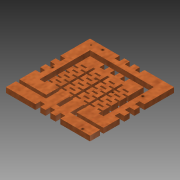
# Autodesk Inventor part: mech
Saved by Autodesk Inventor 2014 SP1 (Build 180222100, 222)
## iProperties
Created: 2015-02-17
Part Number: mech
Material: Wood (Cherry)
Document SubType Name: Modeling
Designer: Erin
Density: 0.63 g/cm^3
Appearance: Cherry - Natural Low Gloss
Author: Erin
Autodesk Inventor part; units mm, degrees
ref_plane "YZ Plane" through (0, 0, 0) normal (1, 0, 0) x (0, 1, 0)
ref_plane "XZ Plane" through (0, 0, 0) normal (0, 1, 0) x (-1, 0, 0)
ref_plane "XY Plane" through (0, 0, 0) normal (0, 0, 1) x (1, 0, 0)
sketch "slots" plane through (0, 0, 0) normal (0, 0, 1) x (1, 0, 0)
  line L0 (61.2067, 31.1821) -> (64.2567, 31.1821)
  line L1 (64.2567, 31.1821) -> (64.2567, 28.1071)
  line L2 (64.2567, 28.1071) -> (61.2067, 28.1071)
  line L3 (61.2067, 28.1071) -> (61.2067, 31.1821)
  line L4 (68.9317, 33.8834) -> (68.9317, 26.9198) construction
  line L5 (67.4067, 31.1821) -> (70.4567, 31.1821)
  line L6 (70.4567, 31.1821) -> (70.4567, 28.1071)
  line L7 (70.4567, 28.1071) -> (67.4067, 28.1071)
  line L8 (67.4067, 28.1071) -> (67.4067, 31.1821)
  line L9 (73.6067, 31.1821) -> (76.6567, 31.1821)
  line L10 (76.6567, 31.1821) -> (76.6567, 28.1071)
  line L11 (76.6567, 28.1071) -> (73.6067, 28.1071)
  line L12 (73.6067, 28.1071) -> (73.6067, 31.1821)
  line L13 (68.9317, 28.1071) -> (68.9317, 27.1937) construction
  point P0 (68.8645, 30.3856)
  dimension "d2" = 3.05
  dimension "d3" = 3.075
  dimension "d99" = 3.15
  dimension "d100" = 3.15
  measures "d2" distance of L1.end L2.end
  measures "d3" distance of L0.end L1.end
  measures "d99" distance between parallel lines of L8 L1
  measures "d100" distance between parallel lines of L12 L6
sketch "flexure" plane through (0, 0, 0) normal (0, 0, 1) x (1, 0, 0)
  line L0 (48.9032, 41.5133) -> (55.9032, 41.5133)
  line L1 (55.9032, 41.5133) -> (55.9032, 19.5133)
  line L2 (55.9032, 19.5133) -> (48.9032, 19.5133)
  line L3 (48.9032, 19.5133) -> (48.9032, 41.5133)
  line L4 (48.9032, 32.2633) -> (51.4486, 32.2633)
  line L5 (51.4486, 32.2633) -> (51.4486, 31.2633)
  line L6 (51.4486, 31.2633) -> (48.9032, 31.2633)
  line L7 (48.9032, 31.2633) -> (48.9032, 32.2633)
  line L8 (53.3577, 31.2633) -> (53.3577, 32.2633)
  line L9 (55.9032, 31.2633) -> (53.3577, 31.2633)
  line L10 (53.3577, 32.2633) -> (55.9032, 32.2633)
  line L11 (55.9032, 32.2633) -> (55.9032, 31.2633)
  line L12 (50.8123, 29.7633) -> (53.9941, 29.7633)
  line L13 (53.9941, 29.7633) -> (53.9941, 28.7633)
  line L14 (53.9941, 28.7633) -> (50.8123, 28.7633)
  line L15 (50.8123, 28.7633) -> (50.8123, 29.7633)
  line L16 (48.9032, 30.5133) -> (55.9032, 30.5133) construction
  line L17 (55.9032, 30.5133) -> (48.9032, 30.5133) construction
  line L18 (53.3577, 27.2633) -> (55.9032, 27.2633)
  line L19 (55.9032, 27.2633) -> (55.9032, 26.2633)
  line L20 (55.9032, 26.2633) -> (53.3577, 26.2633)
  line L21 (53.3577, 26.2633) -> (53.3577, 27.2633)
  line L22 (50.8123, 24.7633) -> (53.9941, 24.7633)
  line L23 (53.9941, 24.7633) -> (53.9941, 23.7633)
  line L24 (53.9941, 23.7633) -> (50.8123, 23.7633)
  line L25 (50.8123, 23.7633) -> (50.8123, 24.7633)
  line L26 (48.9032, 27.2633) -> (51.4486, 27.2633)
  line L27 (51.4486, 27.2633) -> (51.4486, 26.2633)
  line L28 (51.4486, 26.2633) -> (48.9032, 26.2633)
  line L29 (48.9032, 26.2633) -> (48.9032, 27.2633)
  line L30 (48.9032, 25.5133) -> (55.9032, 25.5133) construction
  line L31 (55.9032, 25.5133) -> (48.9032, 25.5133) construction
  line L32 (53.3577, 37.2633) -> (55.9032, 37.2633)
  line L33 (55.9032, 37.2633) -> (55.9032, 36.2633)
  line L34 (55.9032, 36.2633) -> (53.3577, 36.2633)
  line L35 (53.3577, 36.2633) -> (53.3577, 37.2633)
  line L36 (50.8123, 34.7633) -> (53.9941, 34.7633)
  line L37 (53.9941, 34.7633) -> (53.9941, 33.7633)
  line L38 (53.9941, 33.7633) -> (50.8123, 33.7633)
  line L39 (50.8123, 33.7633) -> (50.8123, 34.7633)
  line L40 (48.9032, 37.2633) -> (51.4486, 37.2633)
  line L41 (51.4486, 37.2633) -> (51.4486, 36.2633)
  line L42 (51.4486, 36.2633) -> (48.9032, 36.2633)
  line L43 (48.9032, 36.2633) -> (48.9032, 37.2633)
  line L44 (48.9032, 35.5133) -> (55.9032, 35.5133) construction
  line L45 (55.9032, 35.5133) -> (48.9032, 35.5133) construction
  line L46 (53.3577, 32.2633) -> (55.9032, 32.2633)
  line L47 (55.9032, 32.2633) -> (55.9032, 31.2633)
  line L48 (55.9032, 31.2633) -> (53.3577, 31.2633)
  line L49 (53.3577, 31.2633) -> (53.3577, 32.2633)
  line L50 (50.8123, 29.7633) -> (53.9941, 29.7633)
  line L51 (53.9941, 29.7633) -> (53.9941, 28.7633)
  line L52 (53.9941, 28.7633) -> (50.8123, 28.7633)
  line L53 (50.8123, 28.7633) -> (50.8123, 29.7633)
  line L54 (48.9032, 32.2633) -> (51.4486, 32.2633)
  line L55 (51.4486, 32.2633) -> (51.4486, 31.2633)
  line L56 (51.4486, 31.2633) -> (48.9032, 31.2633)
  line L57 (48.9032, 31.2633) -> (48.9032, 32.2633)
  line L58 (48.9032, 30.5133) -> (55.9032, 30.5133) construction
  line L59 (55.9032, 30.5133) -> (48.9032, 30.5133) construction
  line L60 (53.3577, 22.2633) -> (55.9032, 22.2633)
  line L61 (55.9032, 22.2633) -> (55.9032, 21.2633)
  line L62 (55.9032, 21.2633) -> (53.3577, 21.2633)
  line L63 (53.3577, 21.2633) -> (53.3577, 22.2633)
  line L64 (50.8123, 19.7633) -> (53.9941, 19.7633)
  line L65 (53.9941, 19.7633) -> (53.9941, 18.7633)
  line L66 (53.9941, 18.7633) -> (50.8123, 18.7633)
  line L67 (50.8123, 18.7633) -> (50.8123, 19.7633)
  line L68 (48.9032, 22.2633) -> (51.4486, 22.2633)
  line L69 (51.4486, 22.2633) -> (51.4486, 21.2633)
  line L70 (51.4486, 21.2633) -> (48.9032, 21.2633)
  line L71 (48.9032, 21.2633) -> (48.9032, 22.2633)
  line L72 (48.9032, 20.5133) -> (55.9032, 20.5133) construction
  line L73 (55.9032, 20.5133) -> (48.9032, 20.5133) construction
  line L74 (53.3577, 27.2633) -> (55.9032, 27.2633)
  line L75 (55.9032, 27.2633) -> (55.9032, 26.2633)
  line L76 (55.9032, 26.2633) -> (53.3577, 26.2633)
  line L77 (53.3577, 26.2633) -> (53.3577, 27.2633)
  line L78 (50.8123, 24.7633) -> (53.9941, 24.7633)
  line L79 (53.9941, 24.7633) -> (53.9941, 23.7633)
  line L80 (53.9941, 23.7633) -> (50.8123, 23.7633)
  line L81 (50.8123, 23.7633) -> (50.8123, 24.7633)
  line L82 (48.9032, 27.2633) -> (51.4486, 27.2633)
  line L83 (51.4486, 27.2633) -> (51.4486, 26.2633)
  line L84 (51.4486, 26.2633) -> (48.9032, 26.2633)
  line L85 (48.9032, 26.2633) -> (48.9032, 27.2633)
  line L86 (48.9032, 25.5133) -> (55.9032, 25.5133) construction
  line L87 (55.9032, 25.5133) -> (48.9032, 25.5133) construction
  line L88 (53.3577, 42.2633) -> (55.9032, 42.2633)
  line L89 (55.9032, 42.2633) -> (55.9032, 41.2633)
  line L90 (55.9032, 41.2633) -> (53.3577, 41.2633)
  line L91 (53.3577, 41.2633) -> (53.3577, 42.2633)
  line L92 (50.8123, 39.7633) -> (53.9941, 39.7633)
  line L93 (53.9941, 39.7633) -> (53.9941, 38.7633)
  line L94 (53.9941, 38.7633) -> (50.8123, 38.7633)
  line L95 (50.8123, 38.7633) -> (50.8123, 39.7633)
  line L96 (48.9032, 42.2633) -> (51.4486, 42.2633)
  line L97 (51.4486, 42.2633) -> (51.4486, 41.2633)
  line L98 (51.4486, 41.2633) -> (48.9032, 41.2633)
  line L99 (48.9032, 41.2633) -> (48.9032, 42.2633)
  line L100 (48.9032, 40.5133) -> (55.9032, 40.5133) construction
  line L101 (55.9032, 40.5133) -> (48.9032, 40.5133) construction
  line L102 (53.3577, 37.2633) -> (55.9032, 37.2633)
  line L103 (55.9032, 37.2633) -> (55.9032, 36.2633)
  line L104 (55.9032, 36.2633) -> (53.3577, 36.2633)
  line L105 (53.3577, 36.2633) -> (53.3577, 37.2633)
  line L106 (50.8123, 34.7633) -> (53.9941, 34.7633)
  line L107 (53.9941, 34.7633) -> (53.9941, 33.7633)
  line L108 (53.9941, 33.7633) -> (50.8123, 33.7633)
  line L109 (50.8123, 33.7633) -> (50.8123, 34.7633)
  line L110 (48.9032, 37.2633) -> (51.4486, 37.2633)
  line L111 (51.4486, 37.2633) -> (51.4486, 36.2633)
  line L112 (51.4486, 36.2633) -> (48.9032, 36.2633)
  line L113 (48.9032, 36.2633) -> (48.9032, 37.2633)
  line L114 (48.9032, 35.5133) -> (55.9032, 35.5133) construction
  line L115 (55.9032, 35.5133) -> (48.9032, 35.5133) construction
  line L116 (53.3577, 32.2633) -> (55.9032, 32.2633)
  line L117 (55.9032, 32.2633) -> (55.9032, 31.2633)
  line L118 (55.9032, 31.2633) -> (53.3577, 31.2633)
  line L119 (53.3577, 31.2633) -> (53.3577, 32.2633)
  line L120 (50.8123, 29.7633) -> (53.9941, 29.7633)
  line L121 (53.9941, 29.7633) -> (53.9941, 28.7633)
  line L122 (53.9941, 28.7633) -> (50.8123, 28.7633)
  line L123 (50.8123, 28.7633) -> (50.8123, 29.7633)
  line L124 (48.9032, 32.2633) -> (51.4486, 32.2633)
  line L125 (51.4486, 32.2633) -> (51.4486, 31.2633)
  line L126 (51.4486, 31.2633) -> (48.9032, 31.2633)
  line L127 (48.9032, 31.2633) -> (48.9032, 32.2633)
  line L128 (48.9032, 30.5133) -> (55.9032, 30.5133) construction
  line L129 (55.9032, 30.5133) -> (48.9032, 30.5133) construction
  point P0 (52.8239, 25.8216)
  dimension "d22" = 7
  dimension "d24" = 2.5455
  dimension "d27" = 4.4546
  dimension "d32" = 1.9091
  dimension "d33" = 3.1818
  dimension "d41" = 1
  dimension "d42" = 1
  dimension "d43" = 1.5
  dimension "d93" = 22
  dimension "d106" = 5
  dimension "d109" = 5
  dimension "d115" = 11.75
  measures "d22" distance of L1.end L2.end
  measures "d24" distance of L4.start L4.end
  measures "d27" distance of L6.end L9.end
  measures "d32" distance between parallel lines of L15 L3
  measures "d33" distance of L12.start L12.end
  measures "d41" distance of L4.end L5.end
  measures "d42" distance of L12.end L13.end
  measures "d43" distance between parallel lines of L12 L6
  measures "d93" distance of L0.end L1.end
  measures "d106" distance of L10.start L18.start
  measures "d109" distance of L10.start L32.start
  measures "d115" distance between parallel lines of L12 L0
sketch "Sketch1" plane through (0, 0, 0) normal (0, 0, 1) x (1, 0, 0)
  line L0 (-25, 25) -> (25, 25) construction
  line L1 (25, 25) -> (25, -25) construction
  line L2 (25, -25) -> (-25, -25) construction
  line L3 (-25, -25) -> (-25, 25) construction
  line L4 (-25, -25) -> (25, -25)
  line L5 (25, -25) -> (25, -19)
  line L6 (25, -19) -> (-25, -19)
  line L7 (-25, -19) -> (-25, -25)
  line L8 (0, 33.5916) -> (0, -39.9789) construction
  line L9 (-35.9054, 0) -> (42.6007, 0) construction
  line L10 (-25, 25) -> (25, 25)
  line L11 (25, 25) -> (25, 19)
  line L12 (25, 19) -> (-25, 19)
  line L13 (-25, 19) -> (-25, 25)
  line L14 (-25, 19) -> (-19, 19)
  line L15 (-19, 19) -> (-19, -17)
  line L16 (-19, -17) -> (-25, -17)
  line L17 (-25, -17) -> (-25, 19)
  line L18 (-19, -17) -> (-9, -17)
  line L19 (-9, -17) -> (-9, -11)
  line L20 (-9, -11) -> (-19, -11)
  line L21 (-19, -11) -> (-19, -17)
  line L22 (25, 19) -> (19, 19)
  line L23 (19, 19) -> (19, -17)
  line L24 (19, -17) -> (25, -17)
  line L25 (25, -17) -> (25, 19)
  line L26 (19, -17) -> (9, -17)
  line L27 (9, -17) -> (9, -11)
  line L28 (9, -11) -> (19, -11)
  line L29 (19, -11) -> (19, -17)
  line L30 (-16, 16) -> (16, 16)
  line L31 (16, 16) -> (16, 11)
  line L32 (16, 11) -> (-16, 11)
  line L33 (-16, 11) -> (-16, 16)
  line L34 (-7.2, -11) -> (-1.2, -11)
  line L35 (-1.2, -11) -> (-1.2, -19)
  line L36 (-1.2, -19) -> (-7.2, -19)
  line L37 (-7.2, -19) -> (-7.2, -11)
  line L38 (1.2, -11) -> (7.2, -11)
  line L39 (7.2, -11) -> (7.2, -19)
  line L40 (7.2, -19) -> (1.2, -19)
  line L41 (1.2, -19) -> (1.2, -11)
  line L42 (-68.1542, 16.5688) -> (-29.44, 16.5688) construction
  line L43 (-29.44, 16.5688) -> (-29.44, -5.0786) construction
  line L44 (-29.44, -5.0786) -> (-68.1542, -5.0786) construction
  line L45 (-68.1542, -5.0786) -> (-68.1542, 16.5688) construction
  circle A0 centre (-21.2866, 22) radius 0.5
  line L46 (-7.725, 25) -> (-4.675, 25)
  line L47 (-4.675, 25) -> (-4.675, 21.925)
  line L48 (-4.675, 21.925) -> (-7.725, 21.925)
  line L49 (-7.725, 21.925) -> (-7.725, 25)
  line L50 (0, 27.7013) -> (0, 20.7377) construction
  line L51 (-1.525, 25) -> (1.525, 25)
  line L52 (1.525, 25) -> (1.525, 21.925)
  line L53 (1.525, 21.925) -> (-1.525, 21.925)
  line L54 (-1.525, 21.925) -> (-1.525, 25)
  line L55 (4.675, 25) -> (7.725, 25)
  line L56 (7.725, 25) -> (7.725, 21.925)
  line L57 (7.725, 21.925) -> (4.675, 21.925)
  line L58 (4.675, 21.925) -> (4.675, 25)
  line L59 (0, 21.925) -> (0, 21.0116) construction
  line L60 (-7.725, -21.925) -> (-4.675, -21.925)
  line L61 (-4.675, -21.925) -> (-4.675, -25)
  line L62 (-4.675, -25) -> (-7.725, -25)
  line L63 (-7.725, -25) -> (-7.725, -21.925)
  line L64 (0, -19.2237) -> (0, -26.1873) construction
  line L65 (-1.525, -21.925) -> (1.525, -21.925)
  line L66 (1.525, -21.925) -> (1.525, -25)
  line L67 (1.525, -25) -> (-1.525, -25)
  line L68 (-1.525, -25) -> (-1.525, -21.925)
  line L69 (4.675, -21.925) -> (7.725, -21.925)
  line L70 (7.725, -21.925) -> (7.725, -25)
  line L71 (7.725, -25) -> (4.675, -25)
  line L72 (4.675, -25) -> (4.675, -21.925)
  line L73 (0, -25) -> (0, -25.9134) construction
  line L74 (-25, -7.725) -> (-25, -4.675)
  line L75 (-25, -4.675) -> (-21.925, -4.675)
  line L76 (-21.925, -4.675) -> (-21.925, -7.725)
  line L77 (-21.925, -7.725) -> (-25, -7.725)
  line L78 (-27.7013, 0) -> (-20.7377, 0) construction
  line L79 (-25, -1.525) -> (-25, 1.525)
  line L80 (-25, 1.525) -> (-21.925, 1.525)
  line L81 (-21.925, 1.525) -> (-21.925, -1.525)
  line L82 (-21.925, -1.525) -> (-25, -1.525)
  line L83 (-25, 4.675) -> (-25, 7.725)
  line L84 (-25, 7.725) -> (-21.925, 7.725)
  line L85 (-21.925, 7.725) -> (-21.925, 4.675)
  line L86 (-21.925, 4.675) -> (-25, 4.675)
  line L87 (-21.925, 0) -> (-21.0116, 0) construction
  line L88 (21.925, -7.725) -> (21.925, -4.675)
  line L89 (21.925, -4.675) -> (25, -4.675)
  line L90 (25, -4.675) -> (25, -7.725)
  line L91 (25, -7.725) -> (21.925, -7.725)
  line L92 (19.2237, 0) -> (26.1873, 0) construction
  line L93 (21.925, -1.525) -> (21.925, 1.525)
  line L94 (21.925, 1.525) -> (25, 1.525)
  line L95 (25, 1.525) -> (25, -1.525)
  line L96 (25, -1.525) -> (21.925, -1.525)
  line L97 (21.925, 4.675) -> (21.925, 7.725)
  line L98 (21.925, 7.725) -> (25, 7.725)
  line L99 (25, 7.725) -> (25, 4.675)
  line L100 (25, 4.675) -> (21.925, 4.675)
  line L101 (25, 0) -> (25.9134, 0) construction
  line L102 (-16, 11) -> (-9, 11)
  line L103 (-9, 11) -> (-9, -11)
  line L104 (-9, -11) -> (-16, -11)
  line L105 (-16, -11) -> (-16, 11)
  line L106 (-16, 1.75) -> (-13.4545, 1.75)
  line L107 (-13.4545, 1.75) -> (-13.4545, 0.75)
  line L108 (-13.4545, 0.75) -> (-16, 0.75)
  line L109 (-16, 0.75) -> (-16, 1.75)
  line L110 (-11.5455, 0.75) -> (-11.5455, 1.75)
  line L111 (-9, 0.75) -> (-11.5455, 0.75)
  line L112 (-11.5455, 1.75) -> (-9, 1.75)
  line L113 (-9, 1.75) -> (-9, 0.75)
  line L114 (-14.0909, -0.75) -> (-10.9091, -0.75)
  line L115 (-10.9091, -0.75) -> (-10.9091, -1.75)
  line L116 (-10.9091, -1.75) -> (-14.0909, -1.75)
  line L117 (-14.0909, -1.75) -> (-14.0909, -0.75)
  line L118 (-16, 0) -> (-9, 0) construction
  line L119 (-9, 0) -> (-16, 0) construction
  line L120 (-11.5455, -3.25) -> (-9, -3.25)
  line L121 (-9, -3.25) -> (-9, -4.25)
  line L122 (-9, -4.25) -> (-11.5455, -4.25)
  line L123 (-11.5455, -4.25) -> (-11.5455, -3.25)
  line L124 (-14.0909, -5.75) -> (-10.9091, -5.75)
  line L125 (-10.9091, -5.75) -> (-10.9091, -6.75)
  line L126 (-10.9091, -6.75) -> (-14.0909, -6.75)
  line L127 (-14.0909, -6.75) -> (-14.0909, -5.75)
  line L128 (-16, -3.25) -> (-13.4545, -3.25)
  line L129 (-13.4545, -3.25) -> (-13.4545, -4.25)
  line L130 (-13.4545, -4.25) -> (-16, -4.25)
  line L131 (-16, -4.25) -> (-16, -3.25)
  line L132 (-16, -5) -> (-9, -5) construction
  line L133 (-9, -5) -> (-16, -5) construction
  line L134 (-11.5455, 6.75) -> (-9, 6.75)
  line L135 (-9, 6.75) -> (-9, 5.75)
  line L136 (-9, 5.75) -> (-11.5455, 5.75)
  line L137 (-11.5455, 5.75) -> (-11.5455, 6.75)
  line L138 (-14.0909, 4.25) -> (-10.9091, 4.25)
  line L139 (-10.9091, 4.25) -> (-10.9091, 3.25)
  line L140 (-10.9091, 3.25) -> (-14.0909, 3.25)
  line L141 (-14.0909, 3.25) -> (-14.0909, 4.25)
  line L142 (-16, 6.75) -> (-13.4545, 6.75)
  line L143 (-13.4545, 6.75) -> (-13.4545, 5.75)
  line L144 (-13.4545, 5.75) -> (-16, 5.75)
  line L145 (-16, 5.75) -> (-16, 6.75)
  line L146 (-16, 5) -> (-9, 5) construction
  line L147 (-9, 5) -> (-16, 5) construction
  line L148 (-11.5455, 1.75) -> (-9, 1.75)
  line L149 (-9, 1.75) -> (-9, 0.75)
  line L150 (-9, 0.75) -> (-11.5455, 0.75)
  line L151 (-11.5455, 0.75) -> (-11.5455, 1.75)
  line L152 (-14.0909, -0.75) -> (-10.9091, -0.75)
  line L153 (-10.9091, -0.75) -> (-10.9091, -1.75)
  line L154 (-10.9091, -1.75) -> (-14.0909, -1.75)
  line L155 (-14.0909, -1.75) -> (-14.0909, -0.75)
  line L156 (-16, 1.75) -> (-13.4545, 1.75)
  line L157 (-13.4545, 1.75) -> (-13.4545, 0.75)
  line L158 (-13.4545, 0.75) -> (-16, 0.75)
  line L159 (-16, 0.75) -> (-16, 1.75)
  line L160 (-16, 0) -> (-9, 0) construction
  line L161 (-9, 0) -> (-16, 0) construction
  line L162 (-11.5455, -8.25) -> (-9, -8.25)
  line L163 (-9, -8.25) -> (-9, -9.25)
  line L164 (-9, -9.25) -> (-11.5455, -9.25)
  line L165 (-11.5455, -9.25) -> (-11.5455, -8.25)
  line L166 (-14.0909, -10.75) -> (-10.9091, -10.75)
  line L167 (-10.9091, -10.75) -> (-10.9091, -11.75)
  line L168 (-10.9091, -11.75) -> (-14.0909, -11.75)
  line L169 (-14.0909, -11.75) -> (-14.0909, -10.75)
  line L170 (-16, -8.25) -> (-13.4545, -8.25)
  line L171 (-13.4545, -8.25) -> (-13.4545, -9.25)
  line L172 (-13.4545, -9.25) -> (-16, -9.25)
  line L173 (-16, -9.25) -> (-16, -8.25)
  line L174 (-16, -10) -> (-9, -10) construction
  line L175 (-9, -10) -> (-16, -10) construction
  line L176 (-11.5455, -3.25) -> (-9, -3.25)
  line L177 (-9, -3.25) -> (-9, -4.25)
  line L178 (-9, -4.25) -> (-11.5455, -4.25)
  line L179 (-11.5455, -4.25) -> (-11.5455, -3.25)
  line L180 (-14.0909, -5.75) -> (-10.9091, -5.75)
  line L181 (-10.9091, -5.75) -> (-10.9091, -6.75)
  line L182 (-10.9091, -6.75) -> (-14.0909, -6.75)
  line L183 (-14.0909, -6.75) -> (-14.0909, -5.75)
  line L184 (-16, -3.25) -> (-13.4545, -3.25)
  line L185 (-13.4545, -3.25) -> (-13.4545, -4.25)
  line L186 (-13.4545, -4.25) -> (-16, -4.25)
  line L187 (-16, -4.25) -> (-16, -3.25)
  line L188 (-16, -5) -> (-9, -5) construction
  line L189 (-9, -5) -> (-16, -5) construction
  line L190 (-11.5455, 11.75) -> (-9, 11.75)
  line L191 (-9, 11.75) -> (-9, 10.75)
  line L192 (-9, 10.75) -> (-11.5455, 10.75)
  line L193 (-11.5455, 10.75) -> (-11.5455, 11.75)
  line L194 (-14.0909, 9.25) -> (-10.9091, 9.25)
  line L195 (-10.9091, 9.25) -> (-10.9091, 8.25)
  line L196 (-10.9091, 8.25) -> (-14.0909, 8.25)
  line L197 (-14.0909, 8.25) -> (-14.0909, 9.25)
  line L198 (-16, 11.75) -> (-13.4545, 11.75)
  line L199 (-13.4545, 11.75) -> (-13.4545, 10.75)
  line L200 (-13.4545, 10.75) -> (-16, 10.75)
  line L201 (-16, 10.75) -> (-16, 11.75)
  line L202 (-16, 10) -> (-9, 10) construction
  line L203 (-9, 10) -> (-16, 10) construction
  line L204 (-11.5455, 6.75) -> (-9, 6.75)
  line L205 (-9, 6.75) -> (-9, 5.75)
  line L206 (-9, 5.75) -> (-11.5455, 5.75)
  line L207 (-11.5455, 5.75) -> (-11.5455, 6.75)
  line L208 (-14.0909, 4.25) -> (-10.9091, 4.25)
  line L209 (-10.9091, 4.25) -> (-10.9091, 3.25)
  line L210 (-10.9091, 3.25) -> (-14.0909, 3.25)
  line L211 (-14.0909, 3.25) -> (-14.0909, 4.25)
  line L212 (-16, 6.75) -> (-13.4545, 6.75)
  line L213 (-13.4545, 6.75) -> (-13.4545, 5.75)
  line L214 (-13.4545, 5.75) -> (-16, 5.75)
  line L215 (-16, 5.75) -> (-16, 6.75)
  line L216 (-16, 5) -> (-9, 5) construction
  line L217 (-9, 5) -> (-16, 5) construction
  line L218 (-11.5455, 1.75) -> (-9, 1.75)
  line L219 (-9, 1.75) -> (-9, 0.75)
  line L220 (-9, 0.75) -> (-11.5455, 0.75)
  line L221 (-11.5455, 0.75) -> (-11.5455, 1.75)
  line L222 (-14.0909, -0.75) -> (-10.9091, -0.75)
  line L223 (-10.9091, -0.75) -> (-10.9091, -1.75)
  line L224 (-10.9091, -1.75) -> (-14.0909, -1.75)
  line L225 (-14.0909, -1.75) -> (-14.0909, -0.75)
  line L226 (-16, 1.75) -> (-13.4545, 1.75)
  line L227 (-13.4545, 1.75) -> (-13.4545, 0.75)
  line L228 (-13.4545, 0.75) -> (-16, 0.75)
  line L229 (-16, 0.75) -> (-16, 1.75)
  line L230 (-16, 0) -> (-9, 0) construction
  line L231 (-9, 0) -> (-16, 0) construction
  line L232 (9, 11) -> (16, 11)
  line L233 (16, 11) -> (16, -11)
  line L234 (16, -11) -> (9, -11)
  line L235 (9, -11) -> (9, 11)
  line L236 (9, 1.75) -> (11.5455, 1.75)
  line L237 (11.5455, 1.75) -> (11.5455, 0.75)
  line L238 (11.5455, 0.75) -> (9, 0.75)
  line L239 (9, 0.75) -> (9, 1.75)
  line L240 (13.4545, 0.75) -> (13.4545, 1.75)
  line L241 (16, 0.75) -> (13.4545, 0.75)
  line L242 (13.4545, 1.75) -> (16, 1.75)
  line L243 (16, 1.75) -> (16, 0.75)
  line L244 (10.9091, -0.75) -> (14.0909, -0.75)
  line L245 (14.0909, -0.75) -> (14.0909, -1.75)
  line L246 (14.0909, -1.75) -> (10.9091, -1.75)
  line L247 (10.9091, -1.75) -> (10.9091, -0.75)
  line L248 (9, 0) -> (16, 0) construction
  line L249 (16, 0) -> (9, 0) construction
  line L250 (13.4545, -3.25) -> (16, -3.25)
  line L251 (16, -3.25) -> (16, -4.25)
  line L252 (16, -4.25) -> (13.4545, -4.25)
  line L253 (13.4545, -4.25) -> (13.4545, -3.25)
  line L254 (10.9091, -5.75) -> (14.0909, -5.75)
  line L255 (14.0909, -5.75) -> (14.0909, -6.75)
  line L256 (14.0909, -6.75) -> (10.9091, -6.75)
  line L257 (10.9091, -6.75) -> (10.9091, -5.75)
  line L258 (9, -3.25) -> (11.5455, -3.25)
  line L259 (11.5455, -3.25) -> (11.5455, -4.25)
  line L260 (11.5455, -4.25) -> (9, -4.25)
  line L261 (9, -4.25) -> (9, -3.25)
  line L262 (9, -5) -> (16, -5) construction
  line L263 (16, -5) -> (9, -5) construction
  line L264 (13.4545, 6.75) -> (16, 6.75)
  line L265 (16, 6.75) -> (16, 5.75)
  line L266 (16, 5.75) -> (13.4545, 5.75)
  line L267 (13.4545, 5.75) -> (13.4545, 6.75)
  line L268 (10.9091, 4.25) -> (14.0909, 4.25)
  line L269 (14.0909, 4.25) -> (14.0909, 3.25)
  line L270 (14.0909, 3.25) -> (10.9091, 3.25)
  line L271 (10.9091, 3.25) -> (10.9091, 4.25)
  line L272 (9, 6.75) -> (11.5455, 6.75)
  line L273 (11.5455, 6.75) -> (11.5455, 5.75)
  line L274 (11.5455, 5.75) -> (9, 5.75)
  line L275 (9, 5.75) -> (9, 6.75)
  line L276 (9, 5) -> (16, 5) construction
  line L277 (16, 5) -> (9, 5) construction
  line L278 (13.4545, 1.75) -> (16, 1.75)
  line L279 (16, 1.75) -> (16, 0.75)
  line L280 (16, 0.75) -> (13.4545, 0.75)
  line L281 (13.4545, 0.75) -> (13.4545, 1.75)
  line L282 (10.9091, -0.75) -> (14.0909, -0.75)
  line L283 (14.0909, -0.75) -> (14.0909, -1.75)
  line L284 (14.0909, -1.75) -> (10.9091, -1.75)
  line L285 (10.9091, -1.75) -> (10.9091, -0.75)
  line L286 (9, 1.75) -> (11.5455, 1.75)
  line L287 (11.5455, 1.75) -> (11.5455, 0.75)
  line L288 (11.5455, 0.75) -> (9, 0.75)
  line L289 (9, 0.75) -> (9, 1.75)
  line L290 (9, 0) -> (16, 0) construction
  line L291 (16, 0) -> (9, 0) construction
  line L292 (13.4545, -8.25) -> (16, -8.25)
  line L293 (16, -8.25) -> (16, -9.25)
  line L294 (16, -9.25) -> (13.4545, -9.25)
  line L295 (13.4545, -9.25) -> (13.4545, -8.25)
  line L296 (10.9091, -10.75) -> (14.0909, -10.75)
  line L297 (14.0909, -10.75) -> (14.0909, -11.75)
  line L298 (14.0909, -11.75) -> (10.9091, -11.75)
  line L299 (10.9091, -11.75) -> (10.9091, -10.75)
  line L300 (9, -8.25) -> (11.5455, -8.25)
  line L301 (11.5455, -8.25) -> (11.5455, -9.25)
  line L302 (11.5455, -9.25) -> (9, -9.25)
  line L303 (9, -9.25) -> (9, -8.25)
  line L304 (9, -10) -> (16, -10) construction
  line L305 (16, -10) -> (9, -10) construction
  line L306 (13.4545, -3.25) -> (16, -3.25)
  line L307 (16, -3.25) -> (16, -4.25)
  line L308 (16, -4.25) -> (13.4545, -4.25)
  line L309 (13.4545, -4.25) -> (13.4545, -3.25)
  line L310 (10.9091, -5.75) -> (14.0909, -5.75)
  line L311 (14.0909, -5.75) -> (14.0909, -6.75)
  line L312 (14.0909, -6.75) -> (10.9091, -6.75)
  line L313 (10.9091, -6.75) -> (10.9091, -5.75)
  line L314 (9, -3.25) -> (11.5455, -3.25)
  line L315 (11.5455, -3.25) -> (11.5455, -4.25)
  line L316 (11.5455, -4.25) -> (9, -4.25)
  line L317 (9, -4.25) -> (9, -3.25)
  line L318 (9, -5) -> (16, -5) construction
  line L319 (16, -5) -> (9, -5) construction
  line L320 (13.4545, 11.75) -> (16, 11.75)
  line L321 (16, 11.75) -> (16, 10.75)
  line L322 (16, 10.75) -> (13.4545, 10.75)
  line L323 (13.4545, 10.75) -> (13.4545, 11.75)
  line L324 (10.9091, 9.25) -> (14.0909, 9.25)
  line L325 (14.0909, 9.25) -> (14.0909, 8.25)
  line L326 (14.0909, 8.25) -> (10.9091, 8.25)
  line L327 (10.9091, 8.25) -> (10.9091, 9.25)
  line L328 (9, 11.75) -> (11.5455, 11.75)
  line L329 (11.5455, 11.75) -> (11.5455, 10.75)
  line L330 (11.5455, 10.75) -> (9, 10.75)
  line L331 (9, 10.75) -> (9, 11.75)
  line L332 (9, 10) -> (16, 10) construction
  line L333 (16, 10) -> (9, 10) construction
  line L334 (13.4545, 6.75) -> (16, 6.75)
  line L335 (16, 6.75) -> (16, 5.75)
  line L336 (16, 5.75) -> (13.4545, 5.75)
  line L337 (13.4545, 5.75) -> (13.4545, 6.75)
  line L338 (10.9091, 4.25) -> (14.0909, 4.25)
  line L339 (14.0909, 4.25) -> (14.0909, 3.25)
  line L340 (14.0909, 3.25) -> (10.9091, 3.25)
  line L341 (10.9091, 3.25) -> (10.9091, 4.25)
  line L342 (9, 6.75) -> (11.5455, 6.75)
  line L343 (11.5455, 6.75) -> (11.5455, 5.75)
  line L344 (11.5455, 5.75) -> (9, 5.75)
  line L345 (9, 5.75) -> (9, 6.75)
  line L346 (9, 5) -> (16, 5) construction
  line L347 (16, 5) -> (9, 5) construction
  line L348 (13.4545, 1.75) -> (16, 1.75)
  line L349 (16, 1.75) -> (16, 0.75)
  line L350 (16, 0.75) -> (13.4545, 0.75)
  line L351 (13.4545, 0.75) -> (13.4545, 1.75)
  line L352 (10.9091, -0.75) -> (14.0909, -0.75)
  line L353 (14.0909, -0.75) -> (14.0909, -1.75)
  line L354 (14.0909, -1.75) -> (10.9091, -1.75)
  line L355 (10.9091, -1.75) -> (10.9091, -0.75)
  line L356 (9, 1.75) -> (11.5455, 1.75)
  line L357 (11.5455, 1.75) -> (11.5455, 0.75)
  line L358 (11.5455, 0.75) -> (9, 0.75)
  line L359 (9, 0.75) -> (9, 1.75)
  line L360 (9, 0) -> (16, 0) construction
  line L361 (16, 0) -> (9, 0) construction
  line L362 (0.7, 11) -> (7.7, 11)
  line L363 (7.7, 11) -> (7.7, -11)
  line L364 (7.7, -11) -> (0.7, -11)
  line L365 (0.7, -11) -> (0.7, 11)
  line L366 (0.7, 1.75) -> (3.2455, 1.75)
  line L367 (3.2455, 1.75) -> (3.2455, 0.75)
  line L368 (3.2455, 0.75) -> (0.7, 0.75)
  line L369 (0.7, 0.75) -> (0.7, 1.75)
  line L370 (5.1545, 0.75) -> (5.1545, 1.75)
  line L371 (7.7, 0.75) -> (5.1545, 0.75)
  line L372 (5.1545, 1.75) -> (7.7, 1.75)
  line L373 (7.7, 1.75) -> (7.7, 0.75)
  line L374 (2.6091, -0.75) -> (5.7909, -0.75)
  line L375 (5.7909, -0.75) -> (5.7909, -1.75)
  line L376 (5.7909, -1.75) -> (2.6091, -1.75)
  line L377 (2.6091, -1.75) -> (2.6091, -0.75)
  line L378 (0.7, 0) -> (7.7, 0) construction
  line L379 (7.7, 0) -> (0.7, 0) construction
  line L380 (5.1545, -3.25) -> (7.7, -3.25)
  line L381 (7.7, -3.25) -> (7.7, -4.25)
  line L382 (7.7, -4.25) -> (5.1545, -4.25)
  line L383 (5.1545, -4.25) -> (5.1545, -3.25)
  line L384 (2.6091, -5.75) -> (5.7909, -5.75)
  line L385 (5.7909, -5.75) -> (5.7909, -6.75)
  line L386 (5.7909, -6.75) -> (2.6091, -6.75)
  line L387 (2.6091, -6.75) -> (2.6091, -5.75)
  line L388 (0.7, -3.25) -> (3.2455, -3.25)
  line L389 (3.2455, -3.25) -> (3.2455, -4.25)
  line L390 (3.2455, -4.25) -> (0.7, -4.25)
  line L391 (0.7, -4.25) -> (0.7, -3.25)
  line L392 (0.7, -5) -> (7.7, -5) construction
  line L393 (7.7, -5) -> (0.7, -5) construction
  line L394 (5.1545, 6.75) -> (7.7, 6.75)
  line L395 (7.7, 6.75) -> (7.7, 5.75)
  line L396 (7.7, 5.75) -> (5.1545, 5.75)
  line L397 (5.1545, 5.75) -> (5.1545, 6.75)
  line L398 (2.6091, 4.25) -> (5.7909, 4.25)
  line L399 (5.7909, 4.25) -> (5.7909, 3.25)
  line L400 (5.7909, 3.25) -> (2.6091, 3.25)
  line L401 (2.6091, 3.25) -> (2.6091, 4.25)
  line L402 (0.7, 6.75) -> (3.2455, 6.75)
  line L403 (3.2455, 6.75) -> (3.2455, 5.75)
  line L404 (3.2455, 5.75) -> (0.7, 5.75)
  line L405 (0.7, 5.75) -> (0.7, 6.75)
  line L406 (0.7, 5) -> (7.7, 5) construction
  line L407 (7.7, 5) -> (0.7, 5) construction
  line L408 (5.1545, 1.75) -> (7.7, 1.75)
  line L409 (7.7, 1.75) -> (7.7, 0.75)
  line L410 (7.7, 0.75) -> (5.1545, 0.75)
  line L411 (5.1545, 0.75) -> (5.1545, 1.75)
  line L412 (2.6091, -0.75) -> (5.7909, -0.75)
  line L413 (5.7909, -0.75) -> (5.7909, -1.75)
  line L414 (5.7909, -1.75) -> (2.6091, -1.75)
  line L415 (2.6091, -1.75) -> (2.6091, -0.75)
  line L416 (0.7, 1.75) -> (3.2455, 1.75)
  line L417 (3.2455, 1.75) -> (3.2455, 0.75)
  line L418 (3.2455, 0.75) -> (0.7, 0.75)
  line L419 (0.7, 0.75) -> (0.7, 1.75)
  line L420 (0.7, 0) -> (7.7, 0) construction
  line L421 (7.7, 0) -> (0.7, 0) construction
  line L422 (5.1545, -8.25) -> (7.7, -8.25)
  line L423 (7.7, -8.25) -> (7.7, -9.25)
  line L424 (7.7, -9.25) -> (5.1545, -9.25)
  line L425 (5.1545, -9.25) -> (5.1545, -8.25)
  line L426 (2.6091, -10.75) -> (5.7909, -10.75)
  line L427 (5.7909, -10.75) -> (5.7909, -11.75)
  line L428 (5.7909, -11.75) -> (2.6091, -11.75)
  line L429 (2.6091, -11.75) -> (2.6091, -10.75)
  line L430 (0.7, -8.25) -> (3.2455, -8.25)
  line L431 (3.2455, -8.25) -> (3.2455, -9.25)
  line L432 (3.2455, -9.25) -> (0.7, -9.25)
  line L433 (0.7, -9.25) -> (0.7, -8.25)
  line L434 (0.7, -10) -> (7.7, -10) construction
  line L435 (7.7, -10) -> (0.7, -10) construction
  line L436 (5.1545, -3.25) -> (7.7, -3.25)
  line L437 (7.7, -3.25) -> (7.7, -4.25)
  line L438 (7.7, -4.25) -> (5.1545, -4.25)
  line L439 (5.1545, -4.25) -> (5.1545, -3.25)
  line L440 (2.6091, -5.75) -> (5.7909, -5.75)
  line L441 (5.7909, -5.75) -> (5.7909, -6.75)
  line L442 (5.7909, -6.75) -> (2.6091, -6.75)
  line L443 (2.6091, -6.75) -> (2.6091, -5.75)
  line L444 (0.7, -3.25) -> (3.2455, -3.25)
  line L445 (3.2455, -3.25) -> (3.2455, -4.25)
  line L446 (3.2455, -4.25) -> (0.7, -4.25)
  line L447 (0.7, -4.25) -> (0.7, -3.25)
  line L448 (0.7, -5) -> (7.7, -5) construction
  line L449 (7.7, -5) -> (0.7, -5) construction
  line L450 (5.1545, 11.75) -> (7.7, 11.75)
  line L451 (7.7, 11.75) -> (7.7, 10.75)
  line L452 (7.7, 10.75) -> (5.1545, 10.75)
  line L453 (5.1545, 10.75) -> (5.1545, 11.75)
  line L454 (2.6091, 9.25) -> (5.7909, 9.25)
  line L455 (5.7909, 9.25) -> (5.7909, 8.25)
  line L456 (5.7909, 8.25) -> (2.6091, 8.25)
  line L457 (2.6091, 8.25) -> (2.6091, 9.25)
  line L458 (0.7, 11.75) -> (3.2455, 11.75)
  line L459 (3.2455, 11.75) -> (3.2455, 10.75)
  line L460 (3.2455, 10.75) -> (0.7, 10.75)
  line L461 (0.7, 10.75) -> (0.7, 11.75)
  line L462 (0.7, 10) -> (7.7, 10) construction
  line L463 (7.7, 10) -> (0.7, 10) construction
  line L464 (5.1545, 6.75) -> (7.7, 6.75)
  line L465 (7.7, 6.75) -> (7.7, 5.75)
  line L466 (7.7, 5.75) -> (5.1545, 5.75)
  line L467 (5.1545, 5.75) -> (5.1545, 6.75)
  line L468 (2.6091, 4.25) -> (5.7909, 4.25)
  line L469 (5.7909, 4.25) -> (5.7909, 3.25)
  line L470 (5.7909, 3.25) -> (2.6091, 3.25)
  line L471 (2.6091, 3.25) -> (2.6091, 4.25)
  line L472 (0.7, 6.75) -> (3.2455, 6.75)
  line L473 (3.2455, 6.75) -> (3.2455, 5.75)
  line L474 (3.2455, 5.75) -> (0.7, 5.75)
  line L475 (0.7, 5.75) -> (0.7, 6.75)
  line L476 (0.7, 5) -> (7.7, 5) construction
  line L477 (7.7, 5) -> (0.7, 5) construction
  line L478 (5.1545, 1.75) -> (7.7, 1.75)
  line L479 (7.7, 1.75) -> (7.7, 0.75)
  line L480 (7.7, 0.75) -> (5.1545, 0.75)
  line L481 (5.1545, 0.75) -> (5.1545, 1.75)
  line L482 (2.6091, -0.75) -> (5.7909, -0.75)
  line L483 (5.7909, -0.75) -> (5.7909, -1.75)
  line L484 (5.7909, -1.75) -> (2.6091, -1.75)
  line L485 (2.6091, -1.75) -> (2.6091, -0.75)
  line L486 (0.7, 1.75) -> (3.2455, 1.75)
  line L487 (3.2455, 1.75) -> (3.2455, 0.75)
  line L488 (3.2455, 0.75) -> (0.7, 0.75)
  line L489 (0.7, 0.75) -> (0.7, 1.75)
  line L490 (0.7, 0) -> (7.7, 0) construction
  line L491 (7.7, 0) -> (0.7, 0) construction
  line L492 (-7.7, 11) -> (-0.7, 11)
  line L493 (-0.7, 11) -> (-0.7, -11)
  line L494 (-0.7, -11) -> (-7.7, -11)
  line L495 (-7.7, -11) -> (-7.7, 11)
  line L496 (-7.7, 1.75) -> (-5.1545, 1.75)
  line L497 (-5.1545, 1.75) -> (-5.1545, 0.75)
  line L498 (-5.1545, 0.75) -> (-7.7, 0.75)
  line L499 (-7.7, 0.75) -> (-7.7, 1.75)
  line L500 (-3.2455, 0.75) -> (-3.2455, 1.75)
  line L501 (-0.7, 0.75) -> (-3.2455, 0.75)
  line L502 (-3.2455, 1.75) -> (-0.7, 1.75)
  line L503 (-0.7, 1.75) -> (-0.7, 0.75)
  line L504 (-5.7909, -0.75) -> (-2.6091, -0.75)
  line L505 (-2.6091, -0.75) -> (-2.6091, -1.75)
  line L506 (-2.6091, -1.75) -> (-5.7909, -1.75)
  line L507 (-5.7909, -1.75) -> (-5.7909, -0.75)
  line L508 (-7.7, 0) -> (-0.7, 0) construction
  line L509 (-0.7, 0) -> (-7.7, 0) construction
  line L510 (-3.2455, -3.25) -> (-0.7, -3.25)
  line L511 (-0.7, -3.25) -> (-0.7, -4.25)
  line L512 (-0.7, -4.25) -> (-3.2455, -4.25)
  line L513 (-3.2455, -4.25) -> (-3.2455, -3.25)
  line L514 (-5.7909, -5.75) -> (-2.6091, -5.75)
  line L515 (-2.6091, -5.75) -> (-2.6091, -6.75)
  line L516 (-2.6091, -6.75) -> (-5.7909, -6.75)
  line L517 (-5.7909, -6.75) -> (-5.7909, -5.75)
  line L518 (-7.7, -3.25) -> (-5.1545, -3.25)
  line L519 (-5.1545, -3.25) -> (-5.1545, -4.25)
  line L520 (-5.1545, -4.25) -> (-7.7, -4.25)
  line L521 (-7.7, -4.25) -> (-7.7, -3.25)
  line L522 (-7.7, -5) -> (-0.7, -5) construction
  line L523 (-0.7, -5) -> (-7.7, -5) construction
  line L524 (-3.2455, 6.75) -> (-0.7, 6.75)
  line L525 (-0.7, 6.75) -> (-0.7, 5.75)
  line L526 (-0.7, 5.75) -> (-3.2455, 5.75)
  line L527 (-3.2455, 5.75) -> (-3.2455, 6.75)
  line L528 (-5.7909, 4.25) -> (-2.6091, 4.25)
  line L529 (-2.6091, 4.25) -> (-2.6091, 3.25)
  line L530 (-2.6091, 3.25) -> (-5.7909, 3.25)
  line L531 (-5.7909, 3.25) -> (-5.7909, 4.25)
  line L532 (-7.7, 6.75) -> (-5.1545, 6.75)
  line L533 (-5.1545, 6.75) -> (-5.1545, 5.75)
  line L534 (-5.1545, 5.75) -> (-7.7, 5.75)
  line L535 (-7.7, 5.75) -> (-7.7, 6.75)
  line L536 (-7.7, 5) -> (-0.7, 5) construction
  line L537 (-0.7, 5) -> (-7.7, 5) construction
  line L538 (-3.2455, 1.75) -> (-0.7, 1.75)
  line L539 (-0.7, 1.75) -> (-0.7, 0.75)
  line L540 (-0.7, 0.75) -> (-3.2455, 0.75)
  line L541 (-3.2455, 0.75) -> (-3.2455, 1.75)
  line L542 (-5.7909, -0.75) -> (-2.6091, -0.75)
  line L543 (-2.6091, -0.75) -> (-2.6091, -1.75)
  line L544 (-2.6091, -1.75) -> (-5.7909, -1.75)
  line L545 (-5.7909, -1.75) -> (-5.7909, -0.75)
  line L546 (-7.7, 1.75) -> (-5.1545, 1.75)
  line L547 (-5.1545, 1.75) -> (-5.1545, 0.75)
  line L548 (-5.1545, 0.75) -> (-7.7, 0.75)
  line L549 (-7.7, 0.75) -> (-7.7, 1.75)
  line L550 (-7.7, 0) -> (-0.7, 0) construction
  line L551 (-0.7, 0) -> (-7.7, 0) construction
  line L552 (-3.2455, -8.25) -> (-0.7, -8.25)
  line L553 (-0.7, -8.25) -> (-0.7, -9.25)
  line L554 (-0.7, -9.25) -> (-3.2455, -9.25)
  line L555 (-3.2455, -9.25) -> (-3.2455, -8.25)
  line L556 (-5.7909, -10.75) -> (-2.6091, -10.75)
  line L557 (-2.6091, -10.75) -> (-2.6091, -11.75)
  line L558 (-2.6091, -11.75) -> (-5.7909, -11.75)
  line L559 (-5.7909, -11.75) -> (-5.7909, -10.75)
  line L560 (-7.7, -8.25) -> (-5.1545, -8.25)
  line L561 (-5.1545, -8.25) -> (-5.1545, -9.25)
  line L562 (-5.1545, -9.25) -> (-7.7, -9.25)
  line L563 (-7.7, -9.25) -> (-7.7, -8.25)
  line L564 (-7.7, -10) -> (-0.7, -10) construction
  line L565 (-0.7, -10) -> (-7.7, -10) construction
  line L566 (-3.2455, -3.25) -> (-0.7, -3.25)
  line L567 (-0.7, -3.25) -> (-0.7, -4.25)
  line L568 (-0.7, -4.25) -> (-3.2455, -4.25)
  line L569 (-3.2455, -4.25) -> (-3.2455, -3.25)
  line L570 (-5.7909, -5.75) -> (-2.6091, -5.75)
  line L571 (-2.6091, -5.75) -> (-2.6091, -6.75)
  line L572 (-2.6091, -6.75) -> (-5.7909, -6.75)
  line L573 (-5.7909, -6.75) -> (-5.7909, -5.75)
  line L574 (-7.7, -3.25) -> (-5.1545, -3.25)
  line L575 (-5.1545, -3.25) -> (-5.1545, -4.25)
  line L576 (-5.1545, -4.25) -> (-7.7, -4.25)
  line L577 (-7.7, -4.25) -> (-7.7, -3.25)
  line L578 (-7.7, -5) -> (-0.7, -5) construction
  line L579 (-0.7, -5) -> (-7.7, -5) construction
  line L580 (-3.2455, 11.75) -> (-0.7, 11.75)
  line L581 (-0.7, 11.75) -> (-0.7, 10.75)
  line L582 (-0.7, 10.75) -> (-3.2455, 10.75)
  line L583 (-3.2455, 10.75) -> (-3.2455, 11.75)
  line L584 (-5.7909, 9.25) -> (-2.6091, 9.25)
  line L585 (-2.6091, 9.25) -> (-2.6091, 8.25)
  line L586 (-2.6091, 8.25) -> (-5.7909, 8.25)
  line L587 (-5.7909, 8.25) -> (-5.7909, 9.25)
  line L588 (-7.7, 11.75) -> (-5.1545, 11.75)
  line L589 (-5.1545, 11.75) -> (-5.1545, 10.75)
  line L590 (-5.1545, 10.75) -> (-7.7, 10.75)
  line L591 (-7.7, 10.75) -> (-7.7, 11.75)
  line L592 (-7.7, 10) -> (-0.7, 10) construction
  line L593 (-0.7, 10) -> (-7.7, 10) construction
  line L594 (-3.2455, 6.75) -> (-0.7, 6.75)
  line L595 (-0.7, 6.75) -> (-0.7, 5.75)
  line L596 (-0.7, 5.75) -> (-3.2455, 5.75)
  line L597 (-3.2455, 5.75) -> (-3.2455, 6.75)
  line L598 (-5.7909, 4.25) -> (-2.6091, 4.25)
  line L599 (-2.6091, 4.25) -> (-2.6091, 3.25)
  line L600 (-2.6091, 3.25) -> (-5.7909, 3.25)
  line L601 (-5.7909, 3.25) -> (-5.7909, 4.25)
  line L602 (-7.7, 6.75) -> (-5.1545, 6.75)
  line L603 (-5.1545, 6.75) -> (-5.1545, 5.75)
  line L604 (-5.1545, 5.75) -> (-7.7, 5.75)
  line L605 (-7.7, 5.75) -> (-7.7, 6.75)
  line L606 (-7.7, 5) -> (-0.7, 5) construction
  line L607 (-0.7, 5) -> (-7.7, 5) construction
  line L608 (-3.2455, 1.75) -> (-0.7, 1.75)
  line L609 (-0.7, 1.75) -> (-0.7, 0.75)
  line L610 (-0.7, 0.75) -> (-3.2455, 0.75)
  line L611 (-3.2455, 0.75) -> (-3.2455, 1.75)
  line L612 (-5.7909, -0.75) -> (-2.6091, -0.75)
  line L613 (-2.6091, -0.75) -> (-2.6091, -1.75)
  line L614 (-2.6091, -1.75) -> (-5.7909, -1.75)
  line L615 (-5.7909, -1.75) -> (-5.7909, -0.75)
  line L616 (-7.7, 1.75) -> (-5.1545, 1.75)
  line L617 (-5.1545, 1.75) -> (-5.1545, 0.75)
  line L618 (-5.1545, 0.75) -> (-7.7, 0.75)
  line L619 (-7.7, 0.75) -> (-7.7, 1.75)
  line L620 (-7.7, 0) -> (-0.7, 0) construction
  line L621 (-0.7, 0) -> (-7.7, 0) construction
  line L622 (-7.725, 16) -> (-4.675, 16)
  line L623 (-4.675, 16) -> (-4.675, 12.925)
  line L624 (-4.675, 12.925) -> (-7.725, 12.925)
  line L625 (-7.725, 12.925) -> (-7.725, 16)
  line L626 (0, 18.7013) -> (0, 11.7377) construction
  line L627 (-1.525, 16) -> (1.525, 16)
  line L628 (1.525, 16) -> (1.525, 12.925)
  line L629 (1.525, 12.925) -> (-1.525, 12.925)
  line L630 (-1.525, 12.925) -> (-1.525, 16)
  line L631 (4.675, 16) -> (7.725, 16)
  line L632 (7.725, 16) -> (7.725, 12.925)
  line L633 (7.725, 12.925) -> (4.675, 12.925)
  line L634 (4.675, 12.925) -> (4.675, 16)
  line L635 (0, 12.925) -> (0, 12.0116) construction
  point P0 (0, 0)
  point P1 (0, 25)
  point P2 (25, 0)
  point P3 (0, 16)
  point P4 (-4.2, -11)
  point P5 (-4.2, -11)
  point P6 (4.2, -11)
  point P7 (4.2, -11)
  dimension "d76" = 7
  dimension "d89" = 1.3
  dimension "d90" = 1.3
  dimension "d91" = 1.4
  dimension "d0" = 50
  dimension "d1" = 50
  dimension "d16" = 6
  dimension "d19" = 6
  dimension "d21" = 5
  dimension "d75" = 3
  dimension "d94" = 3
  dimension "d95" = 2
  dimension "d96" = 6
  dimension "d97" = 6
  dimension "d101" = 32
  dimension "d114" = 1
  constraints: 84 end point, 23 horizontal, 20 parallel, 11 perpendicular, 10 vertical, 5 equal length, 5 midpoint, 3 collinear, 2 coincident, 2 point on line, 2 vertical alignment, 1 centre point, 1 horizontal alignment, 4 other
  measures "d0" distance of L1.end L2.end
  measures "d1" distance of L0.end L1.end
  measures "d16" distance between parallel lines of L12 L10
  measures "d19" distance between parallel lines of L4 L6
  measures "d21" distance between parallel lines of L32 L30
  measures "d75" distance between parallel lines of L33 L15
  measures "d94" distance between parallel lines of L30 L12
  measures "d95" distance between parallel lines of L6 L16
  measures "d96" distance of L35.end L36.end
  measures "d97" distance of L39.end L40.end
  measures "d101" distance of L30.start L30.end
  measures "d114" diameter of A0
extrude "Extrusion3" add sketch "Sketch1" along normal blind 3.1 contours L7 L6 L5 L4 L70 L69 L72 L66 L65 L68 L61 L60 L63 | L37 L34 L559 L558 L557 L35 L6 | L494 L495 L562 L561 L560 L520 L519 L518 L498 L497 L496 L534 L533 L532 L590 L589 L32 L583 L582 L493 L524 L527 L526 L502 L500 L501 L510 L513 L512 L552 L555 L554 L34 L557 L556 L559 | L41 L38 L429 L428 L427 L39 L6 | L559 L556 L557 L34 | L34 L557 L558 L559 | L364 L365 L432 L431 L430 L390 L389 L388 L368 L367 L366 L404 L403 L402 L460 L459 L32 L453 L452 L363 L394 L397 L396 L372 L370 L371 L380 L383 L382 L422 L425 L424 L38 L427 L426 L429 | L429 L426 L427 L38 | L38 L427 L428 L429 | L495 L32 L589 L590 | L582 L583 L32 L493 | L591 L588 L589 L32 | L32 L191 L190 L193 L199 L198 L33 L30 L625 L624 L623 L630 L629 L628 L634 L633 L632 L31 L320 L323 L329 L328 L331 L451 L450 L453 L459 L458 L461 L581 L580 L583 L589 L588 L591 | L365 L32 L459 L460 | L32 L583 L580 L581 | L103 L192 L193 L32 | L32 L193 L190 L191 | L452 L453 L32 L363 | L461 L458 L459 L32 | L193 L192 L103 L134 L137 L136 L112 L110 L111 L120 L123 L122 L162 L165 L164 L20 L167 L166 L169 L105 L172 L171 L170 L130 L129 L128 L108 L107 L106 L144 L143 L142 L200 L199 L32 | L32 L453 L450 L451 | L199 L200 L105 L32 | L32 L33 L198 L199 | L331 L328 L329 L32 | L32 L329 L330 L235 | L32 L323 L322 L233 L264 L267 L266 L242 L240 L241 L250 L253 L252 L292 L295 L294 L28 L297 L296 L299 L235 L302 L301 L300 L260 L259 L258 L238 L237 L236 L274 L273 L272 L330 L329 | L323 L320 L31 L32 | L32 L233 L322 L323 | L19 L18 L15 L20 L169 L168 L167 | L167 L168 L169 L20 | L20 L169 L166 L167 | L16 L17 L77 L76 L75 L82 L81 L80 L86 L85 L84 L12 L15 | L28 L299 L298 L297 L23 L26 L27 | L299 L296 L297 L28 | L28 L297 L298 L299 | L12 L13 L10 L49 L48 L47 L54 L53 L52 L58 L57 L56 L11 | L23 L12 L25 L98 L97 L100 L94 L93 L96 L89 L88 L91 L24
equation "\"d2\" = mat - kerf"
equation "\"d3\" = mat - 0.5 * kerf"
equation "\"d22\" = flex_w"
equation "\"d24\" = 0.363636 * flex_w"
equation "\"d27\" = 0.636364 * flex_w"
equation "\"d32\" = 0.272727 * flex_w"
equation "\"d33\" = 0.454545 * flex_w"
equation "\"d41\" = line_w"
equation "\"d42\" = line_w"
equation "\"d43\" = line_sp"
equation "\"d93\" = flex_h"
equation "\"d89\" = flex_sp"
equation "\"d90\" = flex_sp"
equation "\"d16\" = structure_w"
equation "\"d19\" = structure_w"
equation "\"structure_w\" = 6"
equation "\"structure_sp\" = 8"
equation "\"flex_w\" = 7"
equation "\"line_w\" = 1"
equation "\"line_sp\" = 1.5"
equation "\"flex_sp\" = 1.3"
equation "\"mat\" = 3.1"
equation "\"kerf\" = 0.05"
equation "\"flex_h\" = 22"
body "Solid3"
